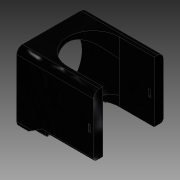
# Autodesk Inventor part: COOLER-HOLDER
Saved by Autodesk Inventor 2014 SP1 (Build 180222100, 222)
## iProperties
Created: 2017-11-29
Part Number: COOLER-HOLDER
Material: Типовые
Document SubType Name: Modeling
Designer: Stepan
Density: 1 g/cm^3
Appearance: Типовые
Author: Stepan
Autodesk Inventor part; units mm, degrees
ref_plane "YZ Plane" through (0, 0, 0) normal (1, 0, 0) x (0, 1, 0)
ref_plane "XZ Plane" through (0, 0, 0) normal (0, 1, 0) x (-1, 0, 0)
ref_plane "XY Plane" through (0, 0, 0) normal (0, 0, 1) x (1, 0, 0)
sketch "Эскиз1" plane through (0, 0, 0) normal (0, 0, 1) x (1, 0, 0)
  line L0 (-15, -15) -> (15, -15)
  line L1 (15, -15) -> (15, 15)
  line L2 (15, 15) -> (-15, 15)
  line L3 (-15, 15) -> (-15, -15)
  line L4 (-15, -15) -> (15, 15) construction
  line L5 (15, -15) -> (-15, 15) construction
  point P0 (0, 0)
  dimension "d0" = 30
  dimension "d1" = 30
  constraints: 12 end point, 2 midpoint, 2 parallel, 1 horizontal, 1 perpendicular
  measures "d0" distance of L2.end L1.end
  measures "d1" distance of L1.end L0.end
extrude "Выдавливание1" add sketch "Эскиз1" against normal blind 26
sketch "Эскиз5" plane through (-15, -15, 0) normal (0, -1, 0) x (1, 0, 0)
  line L0 (30, -26) -> (0, -26) projected
  line L1 (30, 0) -> (30, -26) projected
  line L2 (0, -26) -> (0, -30)
  line L3 (0, -26) -> (6, -26) construction
  line L4 (0, -30) -> (6, -26)
  point P0 (15, 0)
  dimension "d13" = 4
  dimension "d14" = 6
  constraints: 6 end point, 1 parallel, 1 point on line
  measures "d13" distance of L0.end L2.end
  measures "d14" distance of L0.end L3.end
extrude "Выдавливание5" add sketch "Эскиз5" against normal up to surface (30 mm away)
sketch "Эскиз6" plane through (-15, -15, 0) normal (-1, 0, 0) x (0, 0, 1)
  line L0 (0, 30) -> (0, 0) projected
  line L1 (0, 30) -> (-30, 30) projected
  line L2 (-30, 0) -> (-30, 30) projected
  line L3 (0, 0) -> (-30, 0) projected
  point P0 (0, 15)
extrude "Выдавливание6" add sketch "Эскиз6" along normal blind 3
sketch "Эскиз7" plane through (0, 0, 0) normal (0, 0, 1) x (1, 0, 0)
  line L0 (15, -15) -> (15, 15) projected
  circle A0 centre (0, 0) radius 11
  line L1 (0, 11) -> (15, 11)
  line L2 (0, -11) -> (15, -11)
  dimension "d19" = 22
  constraints: 4 end point, 2 point on circle, 2 point on line, 2 tangent, 1 centre point, 1 coincident, 1 parallel, 1 perpendicular
  measures "d19" diameter of A0
extrude "Выдавливание7" cut sketch "Эскиз7" against normal up to next
sketch "Эскиз8" plane through (-18, -15, 0) normal (-1, 0, 0) x (0, 0, 1)
  circle A0 centre (-15, 15) radius 13
  point P0 (0, 15)
  dimension "d22" = 26
  constraints: 1 centre point
  measures "d22" diameter of A0
extrude "Выдавливание8" cut sketch "Эскиз8" against normal blind 18
sketch "Эскиз9" plane through (0, 0, -26) normal (0, 0, -1) x (-1, 0, 0)
  line L0 (9, -15) -> (9, -6.9282) projected
  line L1 (6, -12) -> (12, -12)
  line L2 (12, -12) -> (12, -14)
  line L3 (12, -14) -> (6, -14)
  line L4 (6, -14) -> (6, -12)
  line L5 (6, -12) -> (12, -14) construction
  line L6 (12, -12) -> (6, -14) construction
  point P0 (9, -13)
  dimension "d25" = 6
  dimension "d26" = 2
  constraints: 12 end point, 2 midpoint, 2 parallel, 1 horizontal, 1 perpendicular, 1 point on line
  measures "d25" distance of L2.end L3.end
  measures "d26" distance of L1.end L2.end
extrude "Выдавливание9" add sketch "Эскиз9" along normal blind 2
sketch "Эскиз10" plane through (0, 0, -26) normal (0, 0, -1) x (-1, 0, 0)
  line L0 (9, 6.9282) -> (9, 15) projected
  line L1 (6, 14) -> (12, 14)
  line L2 (12, 14) -> (12, 12)
  line L3 (12, 12) -> (6, 12)
  line L4 (6, 12) -> (6, 14)
  line L5 (6, 14) -> (12, 12) construction
  line L6 (12, 14) -> (6, 12) construction
  point P0 (9, 13)
  dimension "d29" = 6
  dimension "d30" = 2
  constraints: 12 end point, 2 midpoint, 2 parallel, 1 horizontal, 1 perpendicular, 1 point on line
  measures "d29" distance of L2.end L3.end
  measures "d30" distance of L1.end L2.end
extrude "Выдавливание10" add sketch "Эскиз10" along normal blind 2
move faces "Переместить грань2" translate (0, 0.75, 0) faces at (-9, -12, -27.3333)
move faces "Переместить грань3" translate (0, -0.75, 0) faces at (-9, 12, -27.3333)
fillet "Сопряжение1" radius 2.5 4 edges at (-1.5, -15, 0) (-1.5, 15, 0) (-16.5, -15, -30) (-16.5, 15, -30)
fillet "Сопряжение2" radius 0.5 8 edges at (-9, -11.25, -28) (-9, -14, -28) (-9, 14, -28) (-9, 11.25, -28) (-6, 12.625, -28) (-6, -12.625, -28) (-6, 14, -27) (-6, -14, -27)
sketch "Эскиз11" plane through (-9, -15, -26) normal (0, -1, 0) x (1, 0, 0)
  line L0 (21.6444, 10.1638) -> (22.6444, 10.1638)
  line L1 (22.6444, 10.1638) -> (22.6444, 13.1638)
  line L2 (22.6444, 13.1638) -> (21.6444, 13.1638)
  line L3 (21.6444, 13.1638) -> (21.6444, 10.1638)
  line L4 (21.6444, 10.1638) -> (22.6444, 13.1638) construction
  line L5 (22.6444, 10.1638) -> (21.6444, 13.1638) construction
  point P0 (9, 26)
  point P1 (22.1444, 11.6638)
  dimension "d35" = 1
  dimension "d36" = 3
  constraints: 12 end point, 2 midpoint, 2 parallel, 1 horizontal, 1 perpendicular
  measures "d35" distance of L2.end L1.end
  measures "d36" distance of L2.end L0.start
extrude "Выдавливание11" cut sketch "Эскиз11" against normal up to surface (30 mm away)
fillet "Сопряжение3" radius 1.25 2 edges at (3, -15, -26) (3, 15, -26)
sketch "Эскиз12" plane through (-18, -15, 0) normal (-1, 0, 0) x (0, 0, 1)
  arc A0 (-27.5, 30) -> (-30, 27.5) centre (-27.5, 27.5) ccw projected
  arc A1 (-30, 2.5) -> (-27.5, 0) centre (-27.5, 2.5) ccw projected
  arc A2 (-2.5, 0) -> (0, 2.5) centre (-2.5, 2.5) ccw projected
  arc A3 (0, 27.5) -> (-2.5, 30) centre (-2.5, 27.5) ccw projected
  circle A4 centre (-27.5, 27.5) radius 1.5
  circle A5 centre (-27.5, 2.5) radius 1.5
  circle A6 centre (-2.5, 2.5) radius 1.5
  circle A7 centre (-2.5, 27.5) radius 1.5
  point P0 (0, 15)
  dimension "d40" = 3
  dimension "d41" = 3
  dimension "d42" = 3
  dimension "d43" = 3
  constraints: 4 centre point, 4 coincident
  measures "d40" diameter of A4
  measures "d41" diameter of A5
  measures "d42" diameter of A6
  measures "d43" diameter of A7
extrude "Выдавливание12" cut sketch "Эскиз12" against normal blind 3.75
